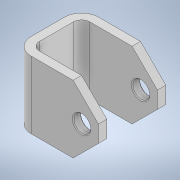
# Autodesk Inventor part: Blacha
Saved by Autodesk Inventor 2021 (Build 250183000, 183)
## iProperties
Created: 2021-05-12
Part Number: Blacha
Material: Ogólny
Document SubType Name: Modeling
Designer: DESKTOP-12
Density: 1 g/cm^3
Appearance: Domyślna
Author: DESKTOP-12
Autodesk Inventor part; units mm, degrees
ref_plane "YZ Plane" through (0, 0, 0) normal (1, 0, 0) x (0, 1, 0)
ref_plane "XZ Plane" through (0, 0, 0) normal (0, 1, 0) x (-1, 0, 0)
ref_plane "XY Plane" through (0, 0, 0) normal (0, 0, 1) x (1, 0, 0)
sketch "Szkic1" plane through (0, 0, 0) normal (0, 1, 0) x (-1, 0, 0)
  line L0 (0, 20) -> (50, 20)
  line L1 (50, 20) -> (50, -20)
  line L2 (50, -20) -> (0, -20)
  line L3 (0, -20) -> (0, -15)
  line L4 (0, -15) -> (45, -15)
  line L5 (45, -15) -> (45, 15)
  line L6 (45, 15) -> (0, 15)
  line L7 (0, 20) -> (0, 15)
  point P0 (0, 0)
  dimension "d0" = 20
  dimension "d1" = 50
  dimension "d2" = 40
  dimension "d3" = 5
  dimension "d5" = 45
  dimension "d6" = 30
  constraints: 16 end point, 3 perpendicular, 1 horizontal, 1 vertical
  measures "d0" distance of point (0, 0) L0.start
  measures "d1" distance of L0.start L0.end
  measures "d2" distance of L0.end L1.end
  measures "d3" distance of L2.end L3.end
  measures "d5" distance of L3.end L4.end
  measures "d6" distance of L4.end L5.end
extrude "Wyciągnięcie proste1" add sketch "Szkic1" along normal blind 40
chamfer "Faza1" distance 15 angle 45 4 edges at (0, 0, -17.5) (0, 40, -17.5) (0, 0, 17.5) (0, 40, 17.5)
fillet "Zaokrąglenie2" radius 10 2 edges at (-50, 20, -20) (-50, 20, 20)
fillet "Zaokrąglenie3" radius 5 2 edges at (-45, 20, -15) (-45, 20, 15)
sketch "Szkic3" plane through (0, 15, 20) normal (0, 0, 1) x (1, 0, 0)
  line L0 (0, 0) -> (0, 10) projected
  line L1 (-40, 25) -> (-15, 25) projected
  point P0 (0, -15)
  point P1 (-10, 5)
  dimension "d35" = 10
  dimension "d36" = 20
  measures "d35" distance from line of L0 point (-10, 5)
  measures "d36" distance from line of L1 point (-10, 5)
hole "Otwór2" at (-10, 20, 20) direction (0, 0, -1) diameter 10 end through all
chamfer "Faza3" distance 0.5 angle 45 4 edges at (-10, 25, 20) (-10, 25, 15) (-10, 25, -20) (-10, 25, -15)
